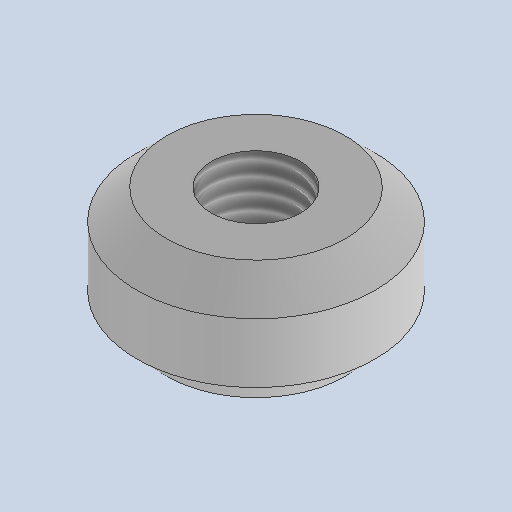
# Autodesk Inventor part: matica
Saved by Autodesk Inventor 2024 (Build 280153000, 153)
## iProperties
Created: 2023-10-02
Part Number: matica
Material: Generic
Document SubType Name: Modeling
Designer: jebes windows
Density: 1 g/cm^3
Appearance: Default
Author: jebes windows
Autodesk Inventor part; units mm, degrees
ref_plane "YZ Plane" through (0, 0, 0) normal (1, 0, 0) x (0, 1, 0)
ref_plane "XZ Plane" through (0, 0, 0) normal (0, 1, 0) x (-1, 0, 0)
ref_plane "XY Plane" through (0, 0, 0) normal (0, 0, 1) x (1, 0, 0)
sketch "Sketch1" plane through (0, 0, 0) normal (0, 0, 1) x (1, 0, 0)
  circle A0 centre (0, 0) radius 1.5 projected
  arc A1 (-3.1429, -28.5256) -> (3.1429, -28.5256) centre (0, -30.9999) ccw projected
  arc A2 (2.5, -26.6698) -> (3.1429, -28.5256) centre (5.5, -26.6698) ccw projected
  line L0 (2.5, -4.3301) -> (2.5, -26.6698) projected
  arc A3 (3.1429, -2.4743) -> (2.5, -4.3301) centre (5.5, -4.3301) ccw projected
  arc A4 (3.1429, -2.4743) -> (-3.1429, -2.4743) centre (0, 0.0001) ccw projected
  arc A5 (-2.5, -4.3301) -> (-3.1429, -2.4743) centre (-5.5, -4.3301) ccw projected
  line L1 (-2.5, -4.3301) -> (-2.5, -26.6698) projected
  arc A6 (-3.1429, -28.5256) -> (-2.5, -26.6698) centre (-5.5, -26.6698) ccw projected
  circle A7 centre (0, -30.9999) radius 1.75 projected
  circle A8 centre (0, 0.0001) radius 1.75 projected
  circle A9 centre (0, 0.0001) radius 4
  circle A10 centre (0, 0.0001) radius 1.4999
  point P0 (0, 0)
  point P1 (-3.1429, -2.4743)
  point P2 (3.1429, -2.4743)
  dimension "d0" = 2.9999
  constraints: 2 centre point, 2 coincident, 1 concentric
  measures "d0" diameter of A10
extrude "Extrusion1" add sketch "Sketch1" against normal blind 4 contours A4 A9 | A8
thread "Thread1" size "M3x0.5" class "6H" standard "ISO Metric profile" length 4
chamfer "Chamfer1" distance 1 angle 45 4 edges at (0, -3.9999, 0) (0, 4.0001, 0) (0, -3.9999, -4) (0, 4.0001, -4)
body "Solid1"
